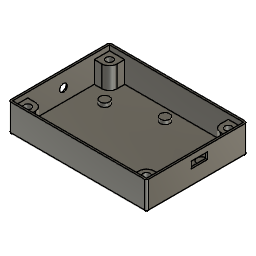
LEDCube Electronics (Autodesk Fusion 360 design; units mm, degrees)
Autodesk Fusion 360 part; units mm, degrees
sketch "Sketch1" plane through (0, 0, 0) normal (0, 0, 1) x (1, 0, 0) in component "Base"
  line L0 (36.25, -26.5) -> (-36.25, -26.5)
  line L1 (-36.25, -26.5) -> (-36.25, 26.5)
  line L2 (-36.25, 26.5) -> (36.25, 26.5)
  line L3 (36.25, 26.5) -> (36.25, -26.5)
  line L4 (36.25, -26.5) -> (-36.25, 26.5) construction
  line L5 (-36.25, -26.5) -> (36.25, 26.5) construction
  dimension "d8" = 72.5
  dimension "d9" = 53
  constraint horizontal L0
  constraint perpendicular L0 L1
  constraint parallel L0 L2
  constraint parallel L1 L3
  constraint coincident L4 origin
  constraint coincident L5 origin
  measures "d8" distance of L1.end L2.end
  measures "d9" distance of L0.end L1.end
extrude "Extrude1" add sketch "Sketch1" along normal blind 15 makes body 1 in component "Base"
shell "Shell1" thickness 1 removed faces 1 at (12.0833, -8.8333, 15) on bodies 1 in component "Base"
sketch "Sketch2" plane through (0, 0, 1) normal (0, 0, 1) x (-1, 0, 0) in component "Base"
  line L0 (-35.25, -25.5) -> (35.25, -25.5)
  line L1 (35.25, -25.5) -> (35.25, 25.5)
  line L2 (35.25, 25.5) -> (-35.25, 25.5)
  line L3 (-35.25, 25.5) -> (-35.25, -25.5)
  circle A0 centre (31.25, -21.5) radius 4
  line L4 (31.25, -17.5) -> (35.25, -17.5)
  line L5 (27.25, -21.5) -> (27.25, -25.5)
  circle A1 centre (31.25, -21.5) radius 1.85
  dimension "d13" = 4
  dimension "d14" = 3.7
  constraint tangent L1 A0
  constraint tangent L0 A0
  constraint coincident A0 L4.start
  constraint coincident L1 L4.end
  constraint tangent A0 L4
  constraint coincident A0 L5.start
  constraint coincident L0 L5.end
  constraint tangent A0 L5
  constraint horizontal L4
  constraint vertical L5
  constraint concentric A0 A1
  measures "d13" radius of A0
  measures "d14" diameter of A1
extrude "Extrude2" add sketch "Sketch2" along normal up to surface (11.3 mm away) contours L0 A0 L5 | L0 L1 A0 | A0 | L1 A0 L4 bodies 1 in component "Base"
mirror "Mirror1" about plane through (0, 0, 0) normal (1, 0, 0) of "Extrude2" in component "Base"
mirror "Mirror2" about plane through (0, 0, 0) normal (0, 1, 0) of "Extrude2", "Mirror1" in component "Base"
sketch "Sketch3" plane through (-36.25, 0, 0) normal (-1, 0, 0) x (0, -1, 0) in component "Base"
  line L0 (-26.5, 0) -> (26.5, 0)
  line L1 (26.5, 0) -> (26.5, 15)
  line L2 (26.5, 15) -> (-26.5, 15)
  line L3 (-26.5, 15) -> (-26.5, 0)
  circle A0 centre (-1.3, 7.5) radius 2
  line L4 (-1.3, 7.5) -> (-1.3, 0) construction
  line L5 (-1.3, 7.5) -> (-26.5, 7.5) construction
  dimension "d25" = 4
  dimension "d73" = 7.5
  dimension "d74" = 25.2
  constraint coincident A0.centre L4.start
  constraint coincident L0 L4.end
  constraint perpendicular L0 L4
  constraint coincident L3 L5.end
  constraint perpendicular L3 L5
  measures "d25" diameter of A0
  measures "d73" distance of A0.centre L4.end
  measures "d74" distance of A0.centre L5.end
extrude "Extrude3" cut sketch "Sketch3" against normal up to surface (1 mm away) contours A0 bodies 1 in component "Base"
sketch "Sketch4" plane through (36.25, 0, 0) normal (1, 0, 0) x (0, 1, 0) in component "Base"
  line L0 (-26.5, 0) -> (26.5, 0)
  line L1 (26.5, 0) -> (26.5, 15)
  line L2 (26.5, 15) -> (-26.5, 15)
  line L3 (-26.5, 15) -> (-26.5, 0)
  line L4 (-3, 12) -> (5.5, 12)
  line L5 (5.5, 12) -> (5.5, 8.5)
  line L6 (5.5, 8.5) -> (-3, 8.5)
  line L7 (-3, 8.5) -> (-3, 12)
  line L8 (-3, 8.5) -> (-26.5, 8.5) construction
  line L9 (-3, 8.5) -> (-3, 0) construction
  dimension "d28" = 8.5
  dimension "d29" = 3.5
  dimension "d31" = 8.5
  dimension "d32" = 23.5
  constraint horizontal L4
  constraint vertical L5
  constraint horizontal L6
  constraint vertical L7
  constraint coincident L3 L8.end
  constraint perpendicular L3 L8
  constraint coincident L0 L9.end
  constraint perpendicular L0 L9
  measures "d28" distance of L4.start L4.end
  measures "d29" distance of L4.start L6.end
  measures "d31" distance of L6.end L9.end
  measures "d32" distance of L6.end L8.end
extrude "Extrude4" cut sketch "Sketch4" against normal up to surface (1 mm away) contours L4 L5 L6 L7 bodies 1 in component "Base"
sketch "Sketch5" plane through (0, 0, 15) normal (0, 0, 1) x (-1, 0, 0) in component "Base"
  line L0 (-35.25, -25.5) -> (-35.25, 25.5)
  line L1 (-35.25, 25.5) -> (35.25, 25.5)
  line L2 (35.25, 25.5) -> (35.25, -25.5)
  line L3 (35.25, -25.5) -> (-35.25, -25.5)
  line L4 (-36.25, -26.5) -> (36.25, -26.5)
  line L5 (36.25, -26.5) -> (36.25, 26.5)
  line L6 (36.25, 26.5) -> (-36.25, 26.5)
  line L7 (-36.25, 26.5) -> (-36.25, -26.5)
extrude "Extrude2'" add sketch "Sketch5" along normal blind 2 separate body contours L0 L1 L2 L3 | L4 L5 L6 L7 makes body 2
copy_body "Body->Comp1" bodies 2 removing the originals makes body 3 in component "Lid (1)"
sketch "Sketch3 (2)" plane through (0, 0, 15) normal (0, 0, -1) x (1, 0, 0)
  line L0 (36.25, -26.5) -> (36.25, 26.5)
  line L1 (36.25, 26.5) -> (-36.25, 26.5)
  line L2 (-36.25, 26.5) -> (-36.25, -26.5)
  line L3 (-36.25, -26.5) -> (36.25, -26.5)
  line L4 (-34.85, -25.1) -> (34.85, -25.1)
  line L5 (34.85, -25.1) -> (34.85, 25.1)
  line L6 (34.85, 25.1) -> (-34.85, 25.1)
  line L7 (-34.85, 25.1) -> (-34.85, -25.1)
  dimension "d42" = -1.4
extrude "Extrude1'" add sketch "Sketch3 (2)" along normal blind 2 contours L4 L5 L6 L7 bodies 3 in component "Lid (1)"
sketch "Sketch3 (3)" plane through (0, 0, 13) normal (0, 0, -1) x (1, 0, 0) in component "Lid (1)"
  line L0 (-34.85, 25.1) -> (-34.85, -25.1)
  line L1 (-34.85, -25.1) -> (34.85, -25.1)
  line L2 (34.85, -25.1) -> (34.85, 25.1)
  line L3 (34.85, 25.1) -> (-34.85, 25.1)
  circle A0 centre (-31.25, 21.5) radius 1.85
  circle A1 centre (-31.25, 21.5) radius 1.7
  dimension "d45" = 3.4
  constraint concentric A0 A1
  measures "d45" diameter of A1
extrude "Extrude2''" cut sketch "Sketch3 (3)" against normal up to surface (4 mm away) contours A1 bodies 3 in component "Lid (1)"
sketch "Sketch4 (2)" plane through (0, 0, 17) normal (0, 0, 1) x (-1, 0, 0) in component "Lid (1)"
  circle A0 centre (31.25, 21.5) radius 1.7
  line L0 (-36.25, 26.5) -> (-36.25, -26.5)
  line L1 (-36.25, -26.5) -> (36.25, -26.5)
  line L2 (36.25, -26.5) -> (36.25, 26.5)
  line L3 (36.25, 26.5) -> (-36.25, 26.5)
  circle A1 centre (31.25, 21.5) radius 3.25
  dimension "d48" = 6.5
  constraint concentric A0 A1
  measures "d48" diameter of A1
extrude "Extrude3'" cut sketch "Sketch4 (2)" against normal blind 2 contours A1 bodies 3 in component "Lid (1)"
mirror "Mirror1'" about plane through (0, 0, 0) normal (0, 1, 0) of "Extrude2''", "Extrude3'" in component "Lid (1)"
mirror "Mirror2'" about plane through (0, 0, 0) normal (1, 0, 0) of "Extrude2''", "Extrude3'", "Mirror1'" in component "Lid (1)"
fillet "Fillet2" radius 1 8 edges at (-36.25, -26.5, 16) (-36.25, 26.5, 16) (0, -26.5, 17) (-36.25, 0, 17) (0, 26.5, 17) (36.25, 26.5, 16) (36.25, 0, 17) (36.25, -26.5, 16) on bodies 3 in component "Lid (1)"
fillet "Fillet3" radius 1 8 edges at (36.25, 26.5, 7.5) (36.25, 0, 0) (0, 26.5, 0) (-36.25, 26.5, 7.5) (-36.25, 0, 0) (-36.25, -26.5, 7.5) (0, -26.5, 0) (36.25, -26.5, 7.5) on bodies 1 in component "Base"
sketch "Sketch5 (2)" plane through (0, 0, 13) normal (0, 0, -1) x (1, 0, 0) in component "Lid (1)"
  circle A0 centre (31.25, -21.5) radius 1.7
  circle A1 centre (31.25, 21.5) radius 1.7
  circle A2 centre (-31.25, -21.5) radius 1.7
  circle A3 centre (-31.25, 21.5) radius 1.7
  line L0 (-34.85, 25.1) -> (-34.85, -25.1)
  line L1 (-34.85, -25.1) -> (34.85, -25.1)
  line L2 (34.85, -25.1) -> (34.85, 25.1)
  line L3 (34.85, 25.1) -> (-34.85, 25.1)
  line L4 (-27.25, 21.5) -> (-27.25, 25.1)
  line L5 (-31.25, 17.5) -> (-34.85, 17.5)
  arc A4 (-31.25, 17.5) -> (-27.25, 21.5) centre (-31.25, 21.5) ccw
  line L6 (20, 0) -> (2.5, 0)
  line L7 (-31.25, -17.5) -> (-34.85, -17.5)
  arc A5 (-27.25, -21.5) -> (-31.25, -17.5) centre (-31.25, -21.5) ccw
  line L8 (-27.25, -21.5) -> (-27.25, -25.1)
  line L9 (0, -2.5) -> (0, -20)
  line L10 (31.25, 17.5) -> (34.85, 17.5)
  arc A6 (27.25, 21.5) -> (31.25, 17.5) centre (31.25, 21.5) ccw
  line L11 (27.25, 21.5) -> (27.25, 25.1)
  line L12 (31.25, -17.5) -> (34.85, -17.5)
  arc A7 (31.25, -17.5) -> (27.25, -21.5) centre (31.25, -21.5) ccw
  line L13 (27.25, -21.5) -> (27.25, -25.1)
  line L14 (34.85, 17.5) -> (34.85, -17.5)
  line L15 (27.25, 25.1) -> (-27.25, 25.1)
  line L16 (-34.85, 17.5) -> (-34.85, -17.5)
  line L17 (-27.25, -25.1) -> (27.25, -25.1)
  line L18 (-26.25, 21.5) -> (-26.25, 24.1)
  line L19 (26.25, 24.1) -> (-26.25, 24.1)
  line L20 (26.25, 21.5) -> (26.25, 24.1)
  arc A8 (26.25, 21.5) -> (31.25, 16.5) centre (31.25, 21.5) ccw
  line L21 (31.25, 16.5) -> (33.85, 16.5)
  line L22 (33.85, 16.5) -> (33.85, -16.5)
  line L23 (31.25, -16.5) -> (33.85, -16.5)
  arc A9 (31.25, -16.5) -> (26.25, -21.5) centre (31.25, -21.5) ccw
  line L24 (26.25, -21.5) -> (26.25, -24.1)
  line L25 (-26.25, -24.1) -> (26.25, -24.1)
  line L26 (-26.25, -21.5) -> (-26.25, -24.1)
  arc A10 (-26.25, -21.5) -> (-31.25, -16.5) centre (-31.25, -21.5) ccw
  line L27 (-31.25, -16.5) -> (-33.85, -16.5)
  line L28 (-33.85, 16.5) -> (-33.85, -16.5)
  line L29 (-31.25, 16.5) -> (-33.85, 16.5)
  arc A11 (-31.25, 16.5) -> (-26.25, 21.5) centre (-31.25, 21.5) ccw
  dimension "d65" = 8
  dimension "d66" = -1
  constraint concentric A3 A4
  constraint coincident L3 L4.end
  constraint tangent L4 A4
  constraint coincident L0 L5.end
  constraint perpendicular L0 L5
  constraint tangent L5 A4
  constraint vertical L4
  constraint symmetric L4.start L6 A5.start
  constraint symmetric L4.end L6 L8.end
  constraint symmetric L5.start L6 L7.start
  constraint symmetric L5.end L6 L7.end
  constraint symmetric A4 L6 A5
  constraint symmetric L4.start L9 A6.start
  constraint symmetric L4.end L9 L11.end
  constraint symmetric L5.start L9 L10.start
  constraint symmetric L5.end L9 L10.end
  constraint symmetric A4 L9 A6
  constraint symmetric L7.start L9 L12.start
  constraint symmetric L7.end L9 L12.end
  constraint symmetric A5.start L9 A7.end
  constraint symmetric A5 L9 A7
  constraint symmetric L8.end L9 L13.end
  measures "d65" diameter of A4
extrude "Extrude4'" cut sketch "Sketch5 (2)" against normal blind 2 contours L18 L19 L20 A8 L21 L22 L23 A9 L24 L25 L26 A10 L27 L28 L29 A11 bodies 3 in component "Lid (1)"
fillet "Fillet3'" radius 0.5 4 edges at (28.2199, 22.6753, 17) (28.2199, -20.3247, 17) (-28.2199, 20.3247, 17) (-28.2199, -22.6753, 17) on bodies 3 in component "Lid (1)"
fillet "Fillet4" radius 0.5 1 edges at (-36.25, 3.1647, 8.2232) on bodies 1 in component "Base"
sketch "Sketch6" plane through (0, 0, 1) normal (0, 0, 1) x (-1, 0, 0) in component "Base"
  line L0 (-31.25, 17.5) -> (-35.25, 17.5)
  line L1 (-35.25, 17.5) -> (-35.25, -17.5)
  line L2 (-35.25, -17.5) -> (-31.25, -17.5)
  arc A0 (-27.25, -21.5) -> (-31.25, -17.5) centre (-31.25, -21.5) ccw
  line L3 (-27.25, -21.5) -> (-27.25, -25.5)
  line L4 (-27.25, -25.5) -> (27.25, -25.5)
  line L5 (27.25, -25.5) -> (27.25, -21.5)
  arc A1 (31.25, -17.5) -> (27.25, -21.5) centre (31.25, -21.5) ccw
  line L6 (31.25, -17.5) -> (35.25, -17.5)
  line L7 (35.25, -17.5) -> (35.25, 17.5)
  line L8 (35.25, 17.5) -> (31.25, 17.5)
  arc A2 (27.25, 21.5) -> (31.25, 17.5) centre (31.25, 21.5) ccw
  line L9 (27.25, 21.5) -> (27.25, 25.5)
  line L10 (27.25, 25.5) -> (-27.25, 25.5)
  line L11 (-27.25, 25.5) -> (-27.25, 21.5)
  arc A3 (-31.25, 17.5) -> (-27.25, 21.5) centre (-31.25, 21.5) ccw
  line L12 (-35.25, -8.9919) -> (-29.75, -8.9919) construction
  circle A4 centre (-29.75, -8.9919) radius 2.5
  line L13 (-29.75, -8.9919) -> (-29.75, -17.7919) construction
  line L14 (0, -25.5) -> (0, -19.5) construction
  circle A5 centre (0, -19.5) radius 2.5
  line L15 (23.75, -25.5) -> (23.75, -11.5) construction
  line L16 (23.75, -11.5) -> (35.25, -11.5) construction
  circle A6 centre (23.75, -11.5) radius 2.5
  line L17 (18.45, 25.5) -> (18.45, 16.4) construction
  line L18 (18.45, 16.4) -> (35.25, 16.4) construction
  circle A7 centre (18.45, 16.4) radius 2.5
  dimension "d77" = 5.5
  dimension "d79" = 5
  dimension "d80" = 8.8
  dimension "d81" = 6
  dimension "d82" = 5
  dimension "d83" = 14
  dimension "d84" = 11.5
  dimension "d85" = 5
  dimension "d86" = 9.1
  dimension "d87" = 16.8
  dimension "d88" = 5
  constraint coincident L1 L12.start
  constraint perpendicular L1 L12
  constraint coincident L12.end A4.centre
  constraint coincident A0 L13.end
  constraint perpendicular L12 L13
  constraint midpoint L4 L14.start
  constraint perpendicular L4 L14
  constraint coincident L14.end A5.centre
  constraint coincident L4 L15.start
  constraint perpendicular L4 L15
  constraint coincident L7 L16.end
  constraint perpendicular L7 L16
  constraint coincident L15.end L16.start
  constraint coincident L10 L17.start
  constraint perpendicular L10 L17
  constraint coincident L7 L18.end
  constraint perpendicular L7 L18
  constraint coincident L17.end L18.start
  measures "d77" distance of L12.start L12.end
  measures "d79" diameter of A4
  measures "d80" distance of L12.end L13.end
  measures "d81" distance of L14.start L14.end
  measures "d82" diameter of A5
  measures "d83" distance of L15.start L15.end
  measures "d84" distance of L15.end L16.end
  measures "d85" diameter of A6
  measures "d86" distance of L17.start L17.end
  measures "d87" distance of L17.end L18.end
  measures "d88" diameter of A7
extrude "Extrude5" add sketch "Sketch6" along normal blind 2 contours A4 | A5 | A6 | A7 bodies 1 in component "Base"
sketch "Sketch1 (2)" plane through (0, 0, 15) normal (0, 0, 1) x (-1, 0, 0) in component "Lid"
  line L0 (-35.25, -25.5) -> (-35.25, 25.5)
  line L1 (-35.25, 25.5) -> (35.25, 25.5)
  line L2 (35.25, 25.5) -> (35.25, -25.5)
  line L3 (35.25, -25.5) -> (-35.25, -25.5)
  line L4 (-36.25, -26.5) -> (36.25, -26.5)
  line L5 (36.25, -26.5) -> (36.25, 26.5)
  line L6 (36.25, 26.5) -> (-36.25, 26.5)
  line L7 (-36.25, 26.5) -> (-36.25, -26.5)
  line L8 (36.25, -26.5) -> (-36.25, -26.5)
  line L9 (-36.25, -26.5) -> (-36.25, 26.5)
  line L10 (-36.25, 26.5) -> (36.25, 26.5)
  line L11 (36.25, 26.5) -> (36.25, -26.5)
  point P0 (36.25, -26.5)
  point P1 (-36.25, 26.5)
  constraint horizontal L8
  constraint vertical L9
  constraint horizontal L10
  constraint vertical L11
  constraint coincident P1 L6.end
  constraint coincident P0 L4.end
extrude "Extrude1''" [suppressed] in component "Lid"
shell "Shell1'" [suppressed] in component "Lid"
component "Base" placed x (1, 0, 0) y (0, 1, 0) z (0, 0, 1) at (0, 0, 0)
component "Lid (1)" placed x (1, 0, 0) y (0, 1, 0) z (0, 0, 1) at (0, 0, 0)
